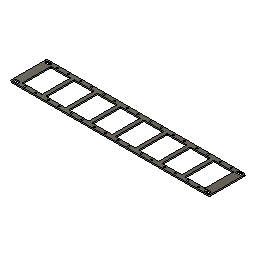
2U 19 Lasercut Bracket (PEM Nut Ready) (Autodesk Fusion 360 design; units mm, degrees)
Autodesk Fusion 360 part; units mm, degrees
sketch "Sketch1" plane through (0, 0, 0) normal (0, 0, 1) x (1, 0, 0) in component "Component"
  line L0 (241.3, 44.5) -> (-241.3, 44.5)
  line L1 (-241.3, 44.5) -> (-241.3, -44.5)
  line L2 (-241.3, -44.5) -> (241.3, -44.5)
  line L3 (241.3, -44.5) -> (241.3, 44.5)
  line L4 (241.3, 44.5) -> (-241.3, -44.5) construction
  line L5 (-241.3, 44.5) -> (241.3, -44.5) construction
  line L6 (-234.3, 34.775) -> (-228.3, 34.775)
  arc A0 (-228.3, 34.775) -> (-228.3, 41.525) centre (-228.3, 38.15) ccw
  line L7 (-228.3, 41.525) -> (-234.3, 41.525)
  arc A1 (-234.3, 41.525) -> (-234.3, 34.775) centre (-234.3, 38.15) ccw
  line L8 (-234.3, 38.15) -> (-228.3, 38.15) construction
  line L9 (-234.3, -41.525) -> (-228.3, -41.525)
  arc A2 (-228.3, -41.525) -> (-228.3, -34.775) centre (-228.3, -38.15) ccw
  line L10 (-228.3, -34.775) -> (-234.3, -34.775)
  arc A3 (-234.3, -34.775) -> (-234.3, -41.525) centre (-234.3, -38.15) ccw
  line L11 (-234.3, -38.15) -> (-228.3, -38.15) construction
  line L12 (0, 0) -> (0, -44.5) construction
  arc A4 (234.3, 34.775) -> (234.3, 41.525) centre (234.3, 38.15) ccw
  line L13 (234.3, 34.775) -> (228.3, 34.775)
  line L14 (228.3, 41.525) -> (234.3, 41.525)
  arc A5 (228.3, 41.525) -> (228.3, 34.775) centre (228.3, 38.15) ccw
  arc A6 (234.3, -41.525) -> (234.3, -34.775) centre (234.3, -38.15) ccw
  line L15 (228.3, -34.775) -> (234.3, -34.775)
  arc A7 (228.3, -34.775) -> (228.3, -41.525) centre (228.3, -38.15) ccw
  line L16 (234.3, -41.525) -> (228.3, -41.525)
  line L17 (-173.3, -34.5) -> (-221.3, -34.5)
  line L18 (-221.3, -34.5) -> (-221.3, 34.5)
  line L19 (-221.3, 34.5) -> (-173.3, 34.5)
  line L20 (-173.3, 34.5) -> (-173.3, -34.5)
  line L21 (-173.3, -34.5) -> (-221.3, 34.5) construction
  line L22 (-221.3, -34.5) -> (-173.3, 34.5) construction
  circle A8 centre (-210.3, 39.5) radius 2.125
  circle A9 centre (-184.3, 39.5) radius 2.125
  circle A10 centre (-210.3, -39.5) radius 2.125
  circle A11 centre (-184.3, -39.5) radius 2.125
  line L23 (-184.3, 39.5) -> (-210.3, 39.5) construction
  line L24 (-197.3, 39.5) -> (-197.3, 34.5) construction
  circle A12 centre (-153.9286, 39.5) radius 2.125
  circle A13 centre (-127.9286, 39.5) radius 2.125
  line L25 (-164.9286, 34.5) -> (-116.9286, 34.5)
  line L26 (-164.9286, -34.5) -> (-164.9286, 34.5)
  line L27 (-116.9286, 34.5) -> (-116.9286, -34.5)
  line L28 (-116.9286, -34.5) -> (-164.9286, -34.5)
  circle A14 centre (-153.9286, -39.5) radius 2.125
  circle A15 centre (-127.9286, -39.5) radius 2.125
  circle A16 centre (-97.5571, 39.5) radius 2.125
  circle A17 centre (-71.5571, 39.5) radius 2.125
  line L29 (-108.5571, 34.5) -> (-60.5571, 34.5)
  line L30 (-108.5571, -34.5) -> (-108.5571, 34.5)
  line L31 (-60.5571, 34.5) -> (-60.5571, -34.5)
  line L32 (-60.5571, -34.5) -> (-108.5571, -34.5)
  circle A18 centre (-97.5571, -39.5) radius 2.125
  circle A19 centre (-71.5571, -39.5) radius 2.125
  circle A20 centre (-41.1857, 39.5) radius 2.125
  circle A21 centre (-15.1857, 39.5) radius 2.125
  line L33 (-52.1857, 34.5) -> (-4.1857, 34.5)
  line L34 (-52.1857, -34.5) -> (-52.1857, 34.5)
  line L35 (-4.1857, 34.5) -> (-4.1857, -34.5)
  line L36 (-4.1857, -34.5) -> (-52.1857, -34.5)
  circle A22 centre (-41.1857, -39.5) radius 2.125
  circle A23 centre (-15.1857, -39.5) radius 2.125
  circle A24 centre (15.1857, 39.5) radius 2.125
  circle A25 centre (41.1857, 39.5) radius 2.125
  line L37 (4.1857, 34.5) -> (52.1857, 34.5)
  line L38 (4.1857, -34.5) -> (4.1857, 34.5)
  line L39 (52.1857, 34.5) -> (52.1857, -34.5)
  line L40 (52.1857, -34.5) -> (4.1857, -34.5)
  circle A26 centre (15.1857, -39.5) radius 2.125
  circle A27 centre (41.1857, -39.5) radius 2.125
  circle A28 centre (71.5571, 39.5) radius 2.125
  circle A29 centre (97.5571, 39.5) radius 2.125
  line L41 (60.5571, 34.5) -> (108.5571, 34.5)
  line L42 (60.5571, -34.5) -> (60.5571, 34.5)
  line L43 (108.5571, 34.5) -> (108.5571, -34.5)
  line L44 (108.5571, -34.5) -> (60.5571, -34.5)
  circle A30 centre (71.5571, -39.5) radius 2.125
  circle A31 centre (97.5571, -39.5) radius 2.125
  circle A32 centre (127.9286, 39.5) radius 2.125
  circle A33 centre (153.9286, 39.5) radius 2.125
  line L45 (116.9286, 34.5) -> (164.9286, 34.5)
  line L46 (116.9286, -34.5) -> (116.9286, 34.5)
  line L47 (164.9286, 34.5) -> (164.9286, -34.5)
  line L48 (164.9286, -34.5) -> (116.9286, -34.5)
  circle A34 centre (127.9286, -39.5) radius 2.125
  circle A35 centre (153.9286, -39.5) radius 2.125
  circle A36 centre (184.3, 39.5) radius 2.125
  circle A37 centre (210.3, 39.5) radius 2.125
  line L49 (173.3, 34.5) -> (221.3, 34.5)
  line L50 (173.3, -34.5) -> (173.3, 34.5)
  line L51 (221.3, 34.5) -> (221.3, -34.5)
  line L52 (221.3, -34.5) -> (173.3, -34.5)
  circle A38 centre (184.3, -39.5) radius 2.125
  circle A39 centre (210.3, -39.5) radius 2.125
  point P0 (-197.3, 0)
  dimension "d1" = 482.6
  dimension "d3" = 6.75
  dimension "d4" = 6
  dimension "d5" = 6.75
  dimension "d6" = 6.35
  dimension "d7" = 7
  dimension "d9" = 6.35
  dimension "d10" = 89
  dimension "d11" = 48
  dimension "d12" = 69
  dimension "d13" = 20
  dimension "d14" = 26
  dimension "d15" = 5
  dimension "d16" = 5
  dimension "d17" = 4.25
  dimension "d20" = 394.6
  dimension "d21" = 0
  constraint horizontal L0
  constraint perpendicular L0 L1
  constraint parallel L0 L2
  constraint parallel L1 L3
  constraint coincident L4 L12.start
  constraint coincident L5 L12.start
  constraint coincident L12.start origin
  constraint tangent L6 A0
  constraint tangent A0 L7
  constraint parallel L6 L7
  constraint tangent L7 A1
  constraint tangent L6 A1
  constraint parallel L0 L8
  constraint tangent L9 A2
  constraint tangent A2 L10
  constraint parallel L9 L10
  constraint tangent L10 A3
  constraint tangent L9 A3
  constraint parallel L2 L11
  constraint vertical A1.centre A3.centre
  constraint vertical A0.centre A2.centre
  constraint midpoint L2 L12.end
  constraint symmetric L6.start L12 A4.start
  constraint symmetric L6.end L12 L13.end
  constraint symmetric A0.end L12 L14.start
  constraint symmetric L7.end L12 A4.end
  constraint symmetric A0 L12 A5
  constraint symmetric A1 L12 A4
  constraint symmetric L9.start L12 A6.start
  constraint symmetric L9.end L12 A7.end
  constraint symmetric A2.end L12 L15.start
  constraint symmetric L10.end L12 A6.end
  constraint symmetric A2 L12 A7
  constraint symmetric A3 L12 A6
  constraint horizontal L17
  constraint perpendicular L17 L18
  constraint parallel L17 L19
  constraint parallel L18 L20
  constraint coincident L21 P0
  constraint coincident L22 P0
  constraint horizontal L12.start P0
  constraint vertical A9.centre A11.centre
  constraint vertical A8.centre A10.centre
  constraint horizontal A8.centre A9.centre
  constraint horizontal A10.centre A11.centre
  constraint coincident A9.centre L23.start
  constraint coincident A8.centre L23.end
  constraint midpoint L23 L24.start
  constraint midpoint L19 L24.end
  constraint vertical L24
  constraint equal A8 A9
  constraint equal A8 A10
  constraint equal A10 A11
  measures "d1" distance of L1.end L2.end
  measures "d3" distance of L6 L7
  measures "d4" distance of A1.centre A0.centre
  measures "d5" distance of L9 L10
  measures "d6" distance of L2 A3.centre
  measures "d7" distance of L1 A3.centre
  measures "d9" distance of L0 A1.centre
  measures "d10" distance of L0.end L1.end
  measures "d11" distance of L18.end L19.end
  measures "d12" distance of L17.end L18.end
  measures "d13" distance of L1 L18
  measures "d14" distance of A8.centre A9.centre
  measures "d15" distance of L0 A8.centre
  measures "d16" distance of L2 A10.centre
  measures "d17" diameter of A8
extrude "Extrude1" add sketch "Sketch1" along normal blind 3.175 in component "Component"
fillet "Fillet1" radius 3 4 edges at (-241.3, -44.5, 1.5875) (-241.3, 44.5, 1.5875) (241.3, 44.5, 1.5875) (241.3, -44.5, 1.5875) in component "Component"
fillet "Fillet1" radius 1 32 edges at (-221.3, 34.5, 1.5875) (-173.3, 34.5, 1.5875) (-164.9286, 34.5, 1.5875) (-116.9286, 34.5, 1.5875) (-108.5571, 34.5, 1.5875) (-52.1857, 34.5, 1.5875) (-60.5571, 34.5, 1.5875) (4.1857, 34.5, 1.5875) (-4.1857, 34.5, 1.5875) (60.5571, 34.5, 1.5875) (52.1857, 34.5, 1.5875) (108.5571, 34.5, 1.5875) (116.9286, 34.5, 1.5875) (173.3, 34.5, 1.5875) (164.9286, 34.5, 1.5875) (221.3, 34.5, 1.5875) (221.3, -34.5, 1.5875) (173.3, -34.5, 1.5875) (164.9286, -34.5, 1.5875) (116.9286, -34.5, 1.5875) (108.5571, -34.5, 1.5875) (60.5571, -34.5, 1.5875) (52.1857, -34.5, 1.5875) (4.1857, -34.5, 1.5875) (-4.1857, -34.5, 1.5875) (-52.1857, -34.5, 1.5875) (-60.5571, -34.5, 1.5875) (-108.5571, -34.5, 1.5875) (-116.9286, -34.5, 1.5875) (-164.9286, -34.5, 1.5875) (-173.3, -34.5, 1.5875) (-221.3, -34.5, 1.5875) in component "Component"
sketch "Sketch2" plane through (0, 0, 3.175) normal (0, 0, 1) x (-1, 0, 0) in component "Component"
  arc A0 (-238.3, 44.5) -> (-241.3, 41.5) centre (-238.3, 41.5) ccw
  line L0 (-241.3, 41.5) -> (-241.3, -41.5)
  arc A1 (-241.3, -41.5) -> (-238.3, -44.5) centre (-238.3, -41.5) ccw
  line L1 (-238.3, -44.5) -> (238.3, -44.5)
  arc A2 (238.3, -44.5) -> (241.3, -41.5) centre (238.3, -41.5) ccw
  line L2 (241.3, -41.5) -> (241.3, 41.5)
  arc A3 (241.3, 41.5) -> (238.3, 44.5) centre (238.3, 41.5) ccw
  line L3 (238.3, 44.5) -> (-238.3, 44.5)
  line L4 (-52.1857, -33.5) -> (-52.1857, 33.5)
  arc A4 (-51.1857, 34.5) -> (-52.1857, 33.5) centre (-51.1857, 33.5) ccw
  line L5 (-51.1857, 34.5) -> (-5.1857, 34.5)
  arc A5 (-4.1857, 33.5) -> (-5.1857, 34.5) centre (-5.1857, 33.5) ccw
  line L6 (-4.1857, 33.5) -> (-4.1857, -33.5)
  arc A6 (-5.1857, -34.5) -> (-4.1857, -33.5) centre (-5.1857, -33.5) ccw
  line L7 (-5.1857, -34.5) -> (-51.1857, -34.5)
  arc A7 (-52.1857, -33.5) -> (-51.1857, -34.5) centre (-51.1857, -33.5) ccw
  circle A8 centre (-15.1857, -39.5) radius 2.125
  circle A9 centre (-15.1857, 39.5) radius 2.125
  circle A10 centre (41.1857, 39.5) radius 2.125
  circle A11 centre (41.1857, -39.5) radius 2.125
  circle A12 centre (-184.3, -39.5) radius 2.125
  circle A13 centre (-210.3, 39.5) radius 2.125
  line L8 (-164.9286, -33.5) -> (-164.9286, 33.5)
  arc A14 (-163.9286, 34.5) -> (-164.9286, 33.5) centre (-163.9286, 33.5) ccw
  line L9 (-163.9286, 34.5) -> (-117.9286, 34.5)
  arc A15 (-116.9286, 33.5) -> (-117.9286, 34.5) centre (-117.9286, 33.5) ccw
  line L10 (-116.9286, 33.5) -> (-116.9286, -33.5)
  arc A16 (-117.9286, -34.5) -> (-116.9286, -33.5) centre (-117.9286, -33.5) ccw
  line L11 (-117.9286, -34.5) -> (-163.9286, -34.5)
  arc A17 (-164.9286, -33.5) -> (-163.9286, -34.5) centre (-163.9286, -33.5) ccw
  circle A18 centre (184.3, -39.5) radius 2.125
  line L12 (220.3, -34.5) -> (174.3, -34.5)
  arc A19 (173.3, -33.5) -> (174.3, -34.5) centre (174.3, -33.5) ccw
  line L13 (173.3, -33.5) -> (173.3, 33.5)
  arc A20 (174.3, 34.5) -> (173.3, 33.5) centre (174.3, 33.5) ccw
  line L14 (174.3, 34.5) -> (220.3, 34.5)
  arc A21 (221.3, 33.5) -> (220.3, 34.5) centre (220.3, 33.5) ccw
  line L15 (221.3, 33.5) -> (221.3, -33.5)
  arc A22 (220.3, -34.5) -> (221.3, -33.5) centre (220.3, -33.5) ccw
  circle A23 centre (127.9286, -39.5) radius 2.125
  circle A24 centre (210.3, 39.5) radius 2.125
  line L16 (4.1857, -33.5) -> (4.1857, 33.5)
  arc A25 (5.1857, 34.5) -> (4.1857, 33.5) centre (5.1857, 33.5) ccw
  line L17 (5.1857, 34.5) -> (51.1857, 34.5)
  arc A26 (52.1857, 33.5) -> (51.1857, 34.5) centre (51.1857, 33.5) ccw
  line L18 (52.1857, 33.5) -> (52.1857, -33.5)
  arc A27 (51.1857, -34.5) -> (52.1857, -33.5) centre (51.1857, -33.5) ccw
  line L19 (51.1857, -34.5) -> (5.1857, -34.5)
  arc A28 (4.1857, -33.5) -> (5.1857, -34.5) centre (5.1857, -33.5) ccw
  circle A29 centre (184.3, 39.5) radius 2.125
  circle A30 centre (210.3, -39.5) radius 2.125
  circle A31 centre (153.9286, -39.5) radius 2.125
  arc A32 (234.3, 34.775) -> (234.3, 41.525) centre (234.3, 38.15) ccw
  line L20 (234.3, 34.775) -> (228.3, 34.775)
  arc A33 (228.3, 41.525) -> (228.3, 34.775) centre (228.3, 38.15) ccw
  line L21 (228.3, 41.525) -> (234.3, 41.525)
  arc A34 (-234.3, -34.775) -> (-234.3, -41.525) centre (-234.3, -38.15) ccw
  line L22 (-234.3, -34.775) -> (-228.3, -34.775)
  arc A35 (-228.3, -41.525) -> (-228.3, -34.775) centre (-228.3, -38.15) ccw
  line L23 (-228.3, -41.525) -> (-234.3, -41.525)
  arc A36 (-228.3, 34.775) -> (-228.3, 41.525) centre (-228.3, 38.15) ccw
  line L24 (-228.3, 34.775) -> (-234.3, 34.775)
  arc A37 (-234.3, 41.525) -> (-234.3, 34.775) centre (-234.3, 38.15) ccw
  line L25 (-234.3, 41.525) -> (-228.3, 41.525)
  arc A38 (234.3, -41.525) -> (234.3, -34.775) centre (234.3, -38.15) ccw
  line L26 (234.3, -41.525) -> (228.3, -41.525)
  arc A39 (228.3, -34.775) -> (228.3, -41.525) centre (228.3, -38.15) ccw
  line L27 (228.3, -34.775) -> (234.3, -34.775)
  circle A40 centre (-153.9286, -39.5) radius 2.125
  circle A41 centre (-184.3, 39.5) radius 2.125
  line L28 (-221.3, -33.5) -> (-221.3, 33.5)
  arc A42 (-220.3, 34.5) -> (-221.3, 33.5) centre (-220.3, 33.5) ccw
  line L29 (-220.3, 34.5) -> (-174.3, 34.5)
  arc A43 (-173.3, 33.5) -> (-174.3, 34.5) centre (-174.3, 33.5) ccw
  line L30 (-173.3, 33.5) -> (-173.3, -33.5)
  arc A44 (-174.3, -34.5) -> (-173.3, -33.5) centre (-174.3, -33.5) ccw
  line L31 (-174.3, -34.5) -> (-220.3, -34.5)
  arc A45 (-221.3, -33.5) -> (-220.3, -34.5) centre (-220.3, -33.5) ccw
  circle A46 centre (-210.3, -39.5) radius 2.125
  circle A47 centre (-127.9286, -39.5) radius 2.125
  circle A48 centre (-127.9286, 39.5) radius 2.125
  circle A49 centre (-153.9286, 39.5) radius 2.125
  line L32 (60.5571, -33.5) -> (60.5571, 33.5)
  arc A50 (61.5571, 34.5) -> (60.5571, 33.5) centre (61.5571, 33.5) ccw
  line L33 (61.5571, 34.5) -> (107.5571, 34.5)
  arc A51 (108.5571, 33.5) -> (107.5571, 34.5) centre (107.5571, 33.5) ccw
  line L34 (108.5571, 33.5) -> (108.5571, -33.5)
  arc A52 (107.5571, -34.5) -> (108.5571, -33.5) centre (107.5571, -33.5) ccw
  line L35 (107.5571, -34.5) -> (61.5571, -34.5)
  arc A53 (60.5571, -33.5) -> (61.5571, -34.5) centre (61.5571, -33.5) ccw
  circle A54 centre (-97.5571, 39.5) radius 2.125
  circle A55 centre (71.5571, 39.5) radius 2.125
  circle A56 centre (-41.1857, -39.5) radius 2.125
  circle A57 centre (-71.5571, -39.5) radius 2.125
  circle A58 centre (97.5571, 39.5) radius 2.125
  line L36 (-108.5571, -33.5) -> (-108.5571, 33.5)
  arc A59 (-107.5571, 34.5) -> (-108.5571, 33.5) centre (-107.5571, 33.5) ccw
  line L37 (-107.5571, 34.5) -> (-61.5571, 34.5)
  arc A60 (-60.5571, 33.5) -> (-61.5571, 34.5) centre (-61.5571, 33.5) ccw
  line L38 (-60.5571, 33.5) -> (-60.5571, -33.5)
  arc A61 (-61.5571, -34.5) -> (-60.5571, -33.5) centre (-61.5571, -33.5) ccw
  line L39 (-61.5571, -34.5) -> (-107.5571, -34.5)
  arc A62 (-108.5571, -33.5) -> (-107.5571, -34.5) centre (-107.5571, -33.5) ccw
  circle A63 centre (-97.5571, -39.5) radius 2.125
  circle A64 centre (-71.5571, 39.5) radius 2.125
  circle A65 centre (15.1857, -39.5) radius 2.125
  circle A66 centre (-41.1857, 39.5) radius 2.125
  circle A67 centre (15.1857, 39.5) radius 2.125
  line L40 (116.9286, -33.5) -> (116.9286, 33.5)
  arc A68 (117.9286, 34.5) -> (116.9286, 33.5) centre (117.9286, 33.5) ccw
  line L41 (117.9286, 34.5) -> (163.9286, 34.5)
  arc A69 (164.9286, 33.5) -> (163.9286, 34.5) centre (163.9286, 33.5) ccw
  line L42 (164.9286, 33.5) -> (164.9286, -33.5)
  arc A70 (163.9286, -34.5) -> (164.9286, -33.5) centre (163.9286, -33.5) ccw
  line L43 (163.9286, -34.5) -> (117.9286, -34.5)
  arc A71 (116.9286, -33.5) -> (117.9286, -34.5) centre (117.9286, -33.5) ccw
  circle A72 centre (153.9286, 39.5) radius 2.125
  circle A73 centre (97.5571, -39.5) radius 2.125
  circle A74 centre (127.9286, 39.5) radius 2.125
  circle A75 centre (71.5571, -39.5) radius 2.125
component "Component" placed x (1, 0, 0) y (0, 1, 0) z (0, 0, 1) at (0, 0, 0)
equation "d5 = d3"
equation "d9 = d6"
equation "d16 = d15"
